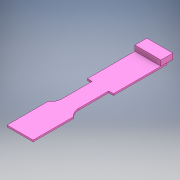
# Autodesk Inventor part: Circuit_center
Saved by Autodesk Inventor 2018 (Build 220112000, 112)
## iProperties
Created: 2018-05-04
Part Number: Circuit_center
Material: Generic
Document SubType Name: Modeling
Designer: suchanek
Density: 1 g/cm^3
Appearance: Default
Author: suchanek
Autodesk Inventor part; units mm, degrees
ref_plane "YZ Plane" through (0, 0, 0) normal (1, 0, 0) x (0, 1, 0)
ref_plane "XZ Plane" through (0, 0, 0) normal (0, 1, 0) x (-1, 0, 0)
ref_plane "XY Plane" through (0, 0, 0) normal (0, 0, 1) x (1, 0, 0)
sketch "Sketch1" plane through (0, 0, 0) normal (0, 0, 1) x (1, 0, 0)
  line L0 (0, 0) -> (16.5, 0)
  line L1 (16.5, 0) -> (16.5, 25.755)
  line L2 (16.5, 85) -> (0, 85)
  line L3 (0, 85) -> (0, 51)
  line L4 (-5, 51) -> (0, 51)
  line L5 (3, 51) -> (3, 32)
  line L6 (-5, 24) -> (-5, 24)
  line L7 (-5, 24) -> (-5, 51)
  arc A0 (-5, 24) -> (0, 25.755) centre (-5, 32) ccw
  line L8 (8.25, 79.5403) -> (8.25, 67.8807)
  line L9 (21.5, 51) -> (16.5, 51)
  line L10 (13.5, 51) -> (13.5, 32)
  line L11 (21.5, 24) -> (21.5, 24)
  line L12 (21.5, 24) -> (21.5, 51)
  arc A1 (13.5, 32) -> (16.5, 25.755) centre (21.5, 32) ccw
  line L13 (0, 51) -> (3, 51)
  line L14 (0, 51) -> (0, 25.755)
  line L15 (0, 25.755) -> (0, 0)
  arc A2 (0, 25.755) -> (3, 32) centre (-5, 32) ccw
  line L16 (16.5, 25.755) -> (16.5, 51)
  arc A3 (16.5, 25.755) -> (21.5, 24) centre (21.5, 32) ccw
  line L17 (16.5, 51) -> (16.5, 85)
  line L18 (16.5, 51) -> (13.5, 51)
  dimension "d0" = 16.5
  dimension "d1" = 85
  dimension "d8" = 8
  dimension "d9" = 3
  dimension "d10" = 19
  dimension "d11" = 32
  constraints: 38 end point, 13 parallel, 8 point on circle, 6 symmetric about line, 5 perpendicular, 4 centre point, 4 horizontal, 3 tangent, 1 point on line, 1 vertical, 2 other
  measures "d0" distance of L0.start L0.end
  measures "d1" distance of L2.end L0.start
  measures "d8" radius of A0
  measures "d9" distance between parallel lines of L5 L3
  measures "d10" distance from line of L4 A0.centre
  measures "d11" distance from line of L0 A0.centre
extrude "Extrusion1" add sketch "Sketch1" along normal blind 1 contours L15 A2 L5 L13 L3 L2 L17 L18 L10 A1 L1 L0
sketch "Sketch2" plane through (0, 0, 1) normal (0, 0, 1) x (1, 0, 0)
  line L0 (-0.005, 81.2) -> (16.505, 81.2)
  line L1 (16.505, 81.2) -> (16.505, 88.8)
  line L2 (16.505, 88.8) -> (-0.005, 88.8)
  line L3 (-0.005, 88.8) -> (-0.005, 81.2)
  line L4 (8.25, 82.8889) -> (8.25, 86.7771)
  line L5 (16.5, 85) -> (0, 85) projected
  line L6 (0, 85) -> (0, 89.9158)
  line L7 (16.5, 85) -> (16.5, 89.26)
  point P0 (0, 0)
  dimension "d4" = 3.8
  dimension "d5" = 16.51
  constraints: 14 end point, 3 vertical, 2 parallel, 1 horizontal, 1 perpendicular, 3 other
  measures "d4" distance between parallel lines of L2 L5
  measures "d5" distance of L1.end L2.end
extrude "Extrusion2" add sketch "Sketch2" along normal blind 3.4
body "Solid1"
